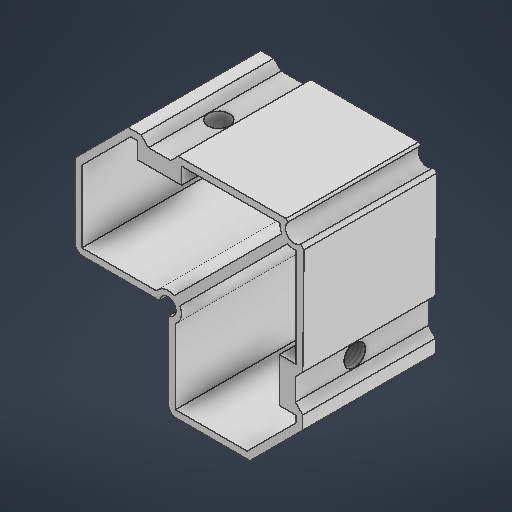
# Autodesk Inventor part: ESCUADRA UNIÓN 45 GORDA
Saved by Autodesk Inventor 2025 (Build 290162000, 162)
## iProperties
Created: 2026-02-05
Part Number: ESCUADRA UNIÓN 45 GORDA
Material: Generic
Document SubType Name: Modeling
Designer: Frank
Density: 1 g/cm^3
Appearance: Default
Author: Frank
Autodesk Inventor part; units mm, degrees
sketch "Sketch1" plane through (0, 0, 0) normal (0, 0, 1) x (1, 0, 0)
  line L0 (0, 0) -> (-27.4191, 0)
  line L1 (-27.4191, 0) -> (-27.4191, -4.6)
  line L2 (-27.4191, -4.6) -> (-39.7191, -4.6)
  line L3 (-39.7191, -4.6) -> (-39.7191, 0)
  line L4 (-39.7191, 0) -> (-41.6191, 0)
  line L5 (-55.1956, -13.5765) -> (-41.6191, 0)
  line L6 (-55.1956, -33.5765) -> (-55.1956, -13.5765)
  line L7 (-34.3956, -33.5765) -> (-55.1956, -33.5765)
  line L8 (1.6418, 1.9) -> (-28.4235, 1.9)
  line L9 (-28.4235, 1.9) -> (-30.4741, -0.1506)
  line L10 (-30.4741, -0.1506) -> (-36.6641, -0.1506)
  line L11 (-36.6641, -0.1506) -> (-38.7147, 1.9)
  line L12 (-42.4061, 1.9) -> (-38.7147, 1.9)
  line L13 (-57.3968, -13.0907) -> (-42.4061, 1.9)
  line L14 (-57.0956, -33.4765) -> (-57.0956, -12.7894)
  line L15 (-33.5097, -35.4765) -> (-55.0956, -35.4765)
  arc A0 (-57.0956, -33.4765) -> (-55.0956, -35.4765) centre (-55.0956, -33.4765) ccw
  line L16 (-29.5043, -32.2942) -> (0.4547, -2.3353)
  line L17 (8.0118, 3.5954) -> (-35.5125, -39.9288) construction
  line L18 (4.4163, -4.4163) -> (4.4163, -31.8354)
  line L19 (4.4163, -31.8354) -> (-0.1837, -31.8354)
  line L20 (-0.1837, -31.8354) -> (-0.1837, -44.1354)
  line L21 (-0.1837, -44.1354) -> (4.4163, -44.1354)
  line L22 (4.4163, -44.1354) -> (4.4163, -46.0354)
  line L23 (-9.1601, -59.6119) -> (4.4163, -46.0354)
  line L24 (-29.1601, -59.6119) -> (-9.1601, -59.6119)
  line L25 (-29.1601, -38.8119) -> (-29.1601, -59.6119)
  line L26 (6.6743, -3.1325) -> (6.3163, -32.8398)
  line L27 (6.3163, -32.8398) -> (4.2657, -34.8904)
  line L28 (4.2657, -34.8904) -> (4.2657, -41.0804)
  line L29 (4.2657, -41.0804) -> (6.3163, -43.131)
  line L30 (6.3163, -46.8224) -> (6.3163, -43.131)
  line L31 (-8.6743, -61.8131) -> (6.3163, -46.8224)
  line L32 (-29.0601, -61.5119) -> (-8.3731, -61.5119)
  line L33 (-31.0601, -37.926) -> (-31.0601, -59.5119)
  arc A1 (-31.0601, -59.5119) -> (-29.0601, -61.5119) centre (-29.0601, -59.5119) ccw
  line L34 (-27.8779, -33.9206) -> (2.081, -3.9617)
  arc A2 (-29.1601, -38.8119) -> (-27.8779, -33.9206) centre (-31.2373, -35.6537) ccw
  arc A3 (-29.5043, -32.2942) -> (-34.3956, -33.5765) centre (-31.2373, -35.6537) ccw
  arc A4 (2.081, -3.9617) -> (4.4163, -4.4163) centre (3.9791, -0.4372) ccw
  arc A5 (0, 0) -> (0.4547, -2.3353) centre (3.9791, -0.4372) ccw
  arc A6 (2.2092, 1.3327) -> (5.749, -2.2072) centre (3.9791, -0.4372) ccw
  arc A7 (-31.0601, -37.926) -> (-33.5097, -35.4765) centre (-31.2373, -35.6537) ccw
  line L35 (1.6418, 1.9) -> (2.2092, 1.3327)
  line L36 (5.749, -2.2072) -> (6.6743, -3.1325)
  point P0 (0, 0)
  point P1 (-57.0956, -35.4765)
  point P2 (-13.7504, -18.1667)
  point P3 (-31.0601, -61.5119)
  point P4 (-29.6257, -34.042)
  dimension "d1" = 4.6
  dimension "d2" = 12.3
  dimension "d3" = 1.9
  dimension "d4" = 135
  dimension "d5" = 19.2
  dimension "d6" = 20
  dimension "d7" = 20.8
  dimension "d10" = 1.9
  dimension "d11" = 2.9
  dimension "d12" = 2.9
  dimension "d14" = 6.19
  dimension "d15" = 3.055
  dimension "d17" = 135
  dimension "d18" = 135
  dimension "d20" = 21.2
  dimension "d22" = 1.9
  dimension "d23" = 1.9
  dimension "d24" = 1.9
  dimension "d25" = 22.687
  dimension "d27" = 2
  dimension "d33" = 2.3
  dimension "d34" = 90
  dimension "d45" = 1.5
  dimension "d46" = 1.5009
  constraints: 74 end point, 21 symmetric about line, 17 point on circle, 10 point on line, 8 centre point, 6 horizontal, 5 parallel, 4 perpendicular, 3 coincident, 2 tangent, 1 collinear, 1 midpoint, 1 vertical, 1 other
  measures "d1" distance of L0.end L1.end
  measures "d2" distance of L1.end L2.end
  measures "d3" distance of L3.end L4.end
  measures "d4" angle of L4 L5
  measures "d5" distance of L5.start L4.end
  measures "d6" distance of L5.start L6.start
  measures "d7" distance of L7.start L6.start
  measures "d10" distance between parallel lines of L8 L0
  measures "d11" distance of L8.end L9.end
  measures "d12" distance of L10.end L11.end
  measures "d14" distance of L9.end L10.end
  measures "d15" distance from line of L3 L10.end
  measures "d17" angle of L8 L9
  measures "d18" angle of L10 L11
  measures "d20" distance of L13.start L12.start
  measures "d22" distance between parallel lines of L14 L6
  measures "d23" distance between parallel lines of L13 L5
  measures "d24" distance between parallel lines of L7 L15
  measures "d25" distance of point (-57.096, -35.476) L14.end
  measures "d27" radius of A0
  measures "d33" distance between parallel lines of L16 L34
  measures "d34" angle of L33 L15
  measures "d45" radial gap between concentric circles of A6 A4
  measures "d46" radial gap between concentric circles of A3 A7
extrude "Extrusion1" add sketch "Sketch1" against normal blind 37
ref_plane "Work Plane1" through (4.2657, -41.0804, 0) normal (1, 0, 0) x (0, 0, -1)
sketch "Sketch2" plane through (4.2657, -41.0804, 0) normal (1, 0, 0) x (0, 0, -1)
  circle A0 centre (16.5, 3.095) radius 3
  line L0 (0, 0) -> (0, 6.19) projected
  line L1 (0, 0) -> (37, 0) projected
  point P0 (0, 41.0804)
  dimension "d52" = 6
  dimension "d53" = 16.5
  dimension "d55" = 3.095
  constraints: 1 centre point
  measures "d52" diameter of A0
  measures "d53" distance from line of L0 A0.centre
  measures "d55" distance from line of L1 A0.centre
extrude "Extrusion2" cut sketch "Sketch2" against normal blind 10
thread "Thread1" size "M6x1" class "6H" standard "ANSI Metric M Profile" full length
ref_plane "Work Plane2" through (-28.6911, -33.1074, 0) normal (0.7071, -0.7071, 0) x (-0.7071, -0.7071, 0)
mirror "Mirror1" about plane through (-28.6911, -33.1074, 0) normal (0.7071, -0.7071, 0) of "Extrusion2"
ref_plane "Plano de trabajo3" through (0, 0, -18.5) normal (0, 0, 1) x (1, 0, 0)
body "Solid1"
